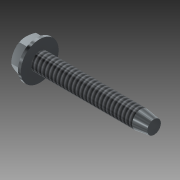
# Autodesk Inventor part: am-1266
Saved by Autodesk Inventor 2018 (Build 220112000, 112)
## iProperties
IsCustomPart: 0
Category: Screw Kit
Company: Autodesk Inc.
Created: 2017-12-13
Part Number: am-1266
Material: Steel, Mild
Description: Plain Indented Hex Washer Head Tapping Screw - Type C - Inch
Document SubType Name: Modeling
Standard: ANSI B18.6.4
Designer: Autodesk Inc.
Standard Revision: 1998
Standards Organization: ANSI
Language: en-US
Size Designation: 10-24 UNC - 1.25
Categories: <MemberInstance><Categories><Category DisplayName="Fasteners" InternalName="e4da775c-781d-43d5-af7c-5136215cf5a6" Mnemonic="FSTN"><Category DisplayName="Bolts" InternalName="536e6df0-f778-49ac-b2f2-25c71d2aa0b2" Mnemonic="SCRW"><CategoryParameter DisplayName="Nominal Diameter" InternalName="8bbe3f8e-44cf-40a9-a251-3a6edc8168d6" Mnemonic="nomdia"/><CategoryParameter DisplayName="Nominal Length" InternalName="238ecbaf-3e6c-45dd-aa95-4068c8e0fd02" Mnemonic="nomlen"/><CategoryParameter DisplayName="Thread Series Designation" InternalName="87c5849c-b3a5-4c3e-9c9b-2feecef9be86" Mnemonic="thrserdsgn"/><CategoryParameter DisplayName="Thread Class" InternalName="ebc0d23b-2cc6-4d2a-b376-d52aae53bab6" Mnemonic="thrclss"/><CategoryParameter DisplayName="Thread Designation" InternalName="586d5e89-370a-4089-914f-0110033585c7" Mnemonic="thrdesign"/><CategoryParameter DisplayName="Thread Type" InternalName="b4bbb7bc-d6aa-4c9f-a9a9-4152b9f6fe49" Mnemonic="thrtype"/><CategoryParameter DisplayName="Threads per Unit" InternalName="bdc6e7d2-ffd0-4d9c-a173-16b95ebb912d" Mnemonic="thrperunit1"/><CategoryParameter DisplayName="Thread Pitch" InternalName="bb82302e-82d8-4176-8fc1-c5d7bb17d5ad" Mnemonic="pitch1"/><CategoryParameter DisplayName="Nominal Diameter Designation" InternalName="03caf894-eafd-4c09-a035-916ac084b87b" Mnemonic="nomdiadesig"/><Category DisplayName="Hex Head - Flanged" InternalName="7925b6b6-1575-406f-8bfa-fe006e82b7bc" Mnemonic="FGPLSCREW"><CategoryParameter DisplayName="Shank Diameter" InternalName="6799ed14-8456-4cfb-bc01-ee9ecb2cdc2b" Mnemonic="grpdia"/><CategoryParameter DisplayName="Grip Length" InternalName="a82b65ac-2d41-4fd1-ba9a-aaa8c8b996d2" Mnemonic="grplen"/><CategoryParameter DisplayName="Thread Length" InternalName="f423544c-1850-46c6-9c68-3a3846636699" Mnemonic="thrlen"/><CategoryParameter DisplayName="Width Across Corners" InternalName="6c4712eb-409b-4c09-a24f-32eb670e2942" Mnemonic="wacor"/><CategoryParameter DisplayName="Head Height" InternalName="5df4f2f2-b824-4910-9115-49166ccd53b4" Mnemonic="headh"/><CategoryParameter DisplayName="Width Across Flats" InternalName="448f2cb5-f593-46ea-8e76-5090215a815d" Mnemonic="waflat"/><CategoryParameter DisplayName="Type" InternalName="851a99d2-714c-4be1-b4b1-e391fdc059ef" Mnemonic="type"/><Category DisplayName="Self Tapping Screws" InternalName="d7140fde-561b-401c-9855-a656e4b6870c" Mnemonic="FLPLCNRGTPSCRW"/></Category></Category></Category><Category DisplayName="DataType" InternalName="23b78d0f-2648-40c6-8793-ca6db495c9e8" Mnemonic="DATATYPE"><CategoryParameter DisplayName="DisplayName" InternalName="05415f3d-3907-474b-a020-eb9d644f4cf3" Mnemonic="DISPLAYNAME"/><CategoryParameter DisplayName="InternalName" InternalName="cf1d0246-76d9-4b4a-8305-fa0409afb5c1" Mnemonic="INTERNALNAME"/><CategoryParameter DisplayName="Folder Name" InternalName="3f06958e-8713-4116-9be7-ed6184ecc97b" Mnemonic="FOLDERNAME"/><CategoryParameter DisplayName="Family Version" InternalName="914462f6-6e19-4b14-ba84-155b9680b1d0" Mnemonic="FAMILYREVISION"/><CategoryParameter DisplayName="ClipFormat" InternalName="bc51e27b-3422-4e78-93ef-cec197ddf230" Mnemonic="CLIPFORMAT"/><CategoryParameter DisplayName="IsMetric" InternalName="e2385c5b-1ea4-4823-96a8-8de651266ec3" Mnemonic="ISMETRIC"/><CategoryParameter DisplayName="Description" InternalName="13903e3d-64b1-4950-80da-f627842ea37f" Mnemonic="DESCRIPTION"/><CategoryParameter DisplayName="StdsOrg" InternalName="8f5914e1-4693-403f-8ab5-d37768198c9d" Mnemonic="STDSORG"/><CategoryParameter DisplayName="Standard" InternalName="0c0a119c-1e12-4c84-803f-101930972f5e" Mnemonic="STANDARD"/><CategoryParameter DisplayName="Manufacturer" InternalName="cd6c7a72-a28a-4e50-99a9-2c7f4e13e5ad" Mnemonic="MANUFACTURER"/><CategoryParameter DisplayName="Member Revision" InternalName="a65d44b9-392f-4f4f-857b-e4b3d54996fe" Mnemonic="MEMBERREVISION"/><CategoryParameter DisplayName="Standard Revision" InternalName="91d5a463-65c2-4fde-b823-3b7fea5e8e17" Mnemonic="STANDARDREVISION"/><CategoryParameter DisplayName="Revision Guid" InternalName="45a75005-10b1-4dfc-8d6d-dfe629f0b93c" Mnemonic="REVISIONGUID"/><CategoryParameter DisplayName="Designation" InternalName="2675968c-4ce5-49e0-a4f5-552d29089031" Mnemonic="DESIGNATION"/><CategoryParameter DisplayName="FileName" InternalName="8b46a4cc-9585-4fed-90c3-899f57e09a73" Mnemonic="FILENAME"/><CategoryParameter DisplayName="Default Row" InternalName="2af9ec52-faaa-4026-b378-f9fa4afca842" Mnemonic="DEFAULTROW"/><Category DisplayName="Part" InternalName="c0e0b642-3bcb-4cc8-9e80-f96d35c4afa4" Mnemonic="PART"><CategoryParameter DisplayName="Material" InternalName="818a152a-d3c3-49ca-80ee-df7d91421b8e" Mnemonic="MATERIAL"/><CategoryParameter DisplayName="Material Key" InternalName="5c9a8adb-dd2b-4535-b97f-0a94a95fe41f" Mnemonic="MATERIALKEY"/><CategoryParameter DisplayName="Part Number" InternalName="016b6077-bfbe-49bd-92c9-d8d59c39c941" Mnemonic="PARTNUMBER"/><CategoryParameter DisplayName="Stock Number" InternalName="4dba7c1c-e26c-444e-836c-b08b433409a8" Mnemonic="STOCKNUMBER"/></Category></Category><Category DisplayName="LegacyMap" InternalName="cd87c42b-3e48-431e-b5c0-1cbeb14dfe77" Mnemonic="LEGACYMAP"><CategoryParameter DisplayName="CatalogName" InternalName="d99d1e27-aa94-4de2-af4c-c348882a6f4f" Mnemonic="CATALOGNAME"/><CategoryParameter DisplayName="FamilyNumber" InternalName="e705e1f4-09cb-413e-91f9-551b4188271e" Mnemonic="FAMILYNUMBER"/><CategoryParameter DisplayName="MemberID" InternalName="8e5e0294-fc51-4c8f-b3d7-003dc5ed94f6" Mnemonic="MEMBERID"/><CategoryParameter DisplayName="unique CC member ID" InternalName="5193edd4-b2b0-4ab4-9d54-de900eee34e0" Mnemonic="CCCOOKIE"/><CategoryParameter DisplayName="unique DA member ID" InternalName="0918ad47-427f-4fed-ae26-24c81c58f590" Mnemonic="DACOOKIE"/><CategoryParameter DisplayName="Merge11 ID" InternalName="0ee8fb18-e2ed-4f39-96f6-1f4b5f50aa71" Mnemonic="MERGE11"/><CategoryParameter DisplayName="Split ID" InternalName="72b5c83c-be7f-45c4-ae51-9160ea6deb26" Mnemonic="SPLIT"/></Category></Categories><FamilyTemplate Id="sh0007"><FamilyTemplateParameters><FamilyTemplateParameter ObjectType="kUserParameterObject" ValueType="xs:double" Id="1" ObjectReferenceKey="KOH"/><FamilyTemplateParameter ObjectType="kUserParameterObject" ValueType="xs:double" Id="2" ObjectReferenceKey="GD2"/><FamilyTemplateParameter ObjectType="kUserParameterObject" ValueType="xs:double" Id="3" ObjectReferenceKey="TPU"/><FamilyTemplateParameter ObjectType="kUserParameterObject" ValueType="xs:double" Id="4" ObjectReferenceKey="SD"/><FamilyTemplateParameter ObjectType="kUserParameterObject" ValueType="xs:double" Id="5" ObjectReferenceKey="GD1"/><FamilyTemplateParameter ObjectType="kUserParameterObject" ValueType="xs:double" Id="6" ObjectReferenceKey="GEL"/><FamilyTemplateParameter ObjectType="kUserParameterObject" ValueType="xs:double" Id="7" ObjectReferenceKey="SW"/><FamilyTemplateParameter ObjectType="kUserParameterObject" ValueType="xs:double" Id="8" ObjectReferenceKey="THREADDIA"/><FamilyTemplateParameter ObjectType="kUserParameterObject" ValueType="xs:double" Id="9" ObjectReferenceKey="TOA"/><FamilyTemplateParameter ObjectType="kUserParameterObject" ValueType="xs:double" Id="10" ObjectReferenceKey="NLG"/><FamilyTemplateParameter ObjectType="kUserParameterObject" ValueType="xs:double" Id="11" ObjectReferenceKey="PTC"/><FamilyTemplateParameter ObjectType="kUserParameterObject" ValueType="xs:double" Id="12" ObjectReferenceKey="NND"/><FamilyTemplateParameter ObjectType="kUserParameterObject" ValueType="xs:double" Id="13" ObjectReferenceKey="SB"/><FamilyTemplateParameter ObjectType="kUserParameterObject" ValueType="xs:double" Id="14" ObjectReferenceKey="SPTZ"/><FamilyTemplateParameter ObjectType="kUserParameterObject" ValueType="xs:double" Id="15" ObjectReferenceKey="SD3"/><FamilyTemplateParameter ObjectType="kUserParameterObject" ValueType="xs:double" Id="16" ObjectReferenceKey="SD2"/><FamilyTemplateParameter ObjectType="kUserParameterObject" ValueType="xs:double" Id="17" ObjectReferenceKey="E0"/><FamilyTemplateParameter ObjectType="kPropertyObject" ValueType="xs:string" Id="100" ObjectReferenceKey="{32853F0F-3444-11d1-9E93-0060B03C1CA6}" SubObjectId="52"/><FamilyTemplateParameter ObjectType="kPropertyObject" ValueType="xs:string" Id="105" ObjectReferenceKey="{32853F0F-3444-11d1-9E93-0060B03C1CA6}" SubObjectId="5"/><FamilyTemplateParameter ObjectType="kPartComponentDefinitionObject" ValueType="xs:string" Id="110" SubObjectId="Material"/><FamilyTemplateParameter ObjectType="kThreadFeatureObject" ValueType="xs:structure" Id="300" ObjectReferenceKey="1002000010000000ad200000000000008000000000000000" SubObjectId="ThreadInfo"><FamilyTemplateParameter ObjectType="" ValueType="xs:string" Id="301" SubObjectId="ThreadDesignation"/><FamilyTemplateParameter ObjectType="" ValueType="xs:string" Id="302" SubObjectId="ThreadType"/><FamilyTemplateParameter ObjectType="" ValueType="xs:string" Id="303" SubObjectId="ThreadClass"/></FamilyTemplateParameter></FamilyTemplateParameters></FamilyTemplate><CategoryParameterMap><ParamToTemplateMap><ParamToTemplate CategoryParameter="//CategoryParameter[@InternalName='05415f3d-3907-474b-a020-eb9d644f4cf3']" ConstantValue="Plain Indented Hex Washer Head Tapping Screw - Type C - Inch"/><ParamToTemplate CategoryParameter="//CategoryParameter[@InternalName='cf1d0246-76d9-4b4a-8305-fa0409afb5c1']" ConstantValue="d649e813-dc5c-4466-8ee0-86f1dc2aa72b"/><ParamToTemplate CategoryParameter="//CategoryParameter[@InternalName='3f06958e-8713-4116-9be7-ed6184ecc97b']" ConstantValue="ANSI B18.6.4(232)"/><ParamToTemplate CategoryParameter="//CategoryParameter[@InternalName='914462f6-6e19-4b14-ba84-155b9680b1d0']" ConstantValue="10"/><ParamToTemplate CategoryParameter="//CategoryParameter[@InternalName='bc51e27b-3422-4e78-93ef-cec197ddf230']" ConstantValue="CF_INVENTOR.STDPARTS"/><ParamToTemplate CategoryParameter="//CategoryParameter[@InternalName='e2385c5b-1ea4-4823-96a8-8de651266ec3']" ConstantValue="false"/><ParamToTemplate CategoryParameter="//CategoryParameter[@InternalName='13903e3d-64b1-4950-80da-f627842ea37f']" ConstantValue="Plain Indented Hex Washer Head Tapping Screw - Type C - Inch"/><ParamToTemplate CategoryParameter="//CategoryParameter[@InternalName='8f5914e1-4693-403f-8ab5-d37768198c9d']" ConstantValue="ANSI"/><ParamToTemplate CategoryParameter="//CategoryParameter[@InternalName='0c0a119c-1e12-4c84-803f-101930972f5e']" ConstantValue="ANSI B18.6.4"/><ParamToTemplate CategoryParameter="//CategoryParameter[@InternalName='cd6c7a72-a28a-4e50-99a9-2c7f4e13e5ad']" TemplateParameter="104"/><ParamToTemplate CategoryParameter="//CategoryParameter[@InternalName='91d5a463-65c2-4fde-b823-3b7fea5e8e17']" ConstantValue="1998"/><ParamToTemplate CategoryParameter="//CategoryParameter[@InternalName='45a75005-10b1-4dfc-8d6d-dfe629f0b93c']" ConstantValue="daae674b-f34b-45e6-9f46-31a5b4692541"/><ParamToTemplate CategoryParameter="//CategoryParameter[@InternalName='2af9ec52-faaa-4026-b378-f9fa4afca842']" ConstantValue="10"/><ParamToTemplate CategoryParameter="//CategoryParameter[@InternalName='d99d1e27-aa94-4de2-af4c-c348882a6f4f']" ConstantValue="ANSI"/><ParamToTemplate CategoryParameter="//CategoryParameter[@InternalName='e705e1f4-09cb-413e-91f9-551b4188271e']" ConstantValue="902"/><ParamToTemplate CategoryParameter="//CategoryParameter[@InternalName='8b46a4cc-9585-4fed-90c3-899f57e09a73']" ConstantValue="ANSI B18.6.4 - 10-24 UNC - 1.25(17) C"/><ParamToTemplate CategoryParameter="//CategoryParameter[@InternalName='a65d44b9-392f-4f4f-857b-e4b3d54996fe']" ConstantValue="4d9bfe0b-fef6-4d20-a557-dd97682ee487"/><ParamToTemplate CategoryParameter="//CategoryParameter[@InternalName='6799ed14-8456-4cfb-bc01-ee9ecb2cdc2b']" ConstantValue="0.19"/><ParamToTemplate CategoryParameter="//CategoryParameter[@InternalName='a82b65ac-2d41-4fd1-ba9a-aaa8c8b996d2']" ConstantValue="0"/><ParamToTemplate CategoryParameter="//CategoryParameter[@InternalName='5df4f2f2-b824-4910-9115-49166ccd53b4']" ConstantValue="0.151"/><ParamToTemplate CategoryParameter="//CategoryParameter[@InternalName='ebc0d23b-2cc6-4d2a-b376-d52aae53bab6']" ConstantValue="2A"/><ParamToTemplate CategoryParameter="//CategoryParameter[@InternalName='b4bbb7bc-d6aa-4c9f-a9a9-4152b9f6fe49']" ConstantValue="ANSI Unified Screw Threads"/><ParamToTemplate CategoryParameter="//CategoryParameter[@InternalName='8e5e0294-fc51-4c8f-b3d7-003dc5ed94f6']" ConstantValue="790"/><ParamToTemplate CategoryParameter="//CategoryParameter[@InternalName='2675968c-4ce5-49e0-a4f5-552d29089031']" TemplateParameter="100"/><ParamToTemplate CategoryParameter="//CategoryParameter[@InternalName='6c4712eb-409b-4c09-a24f-32eb670e2942']" TemplateParameter="17"/><ParamToTemplate CategoryParameter="//CategoryParameter[@InternalName='f423544c-1850-46c6-9c68-3a3846636699']" TemplateParameter="6"/><ParamToTemplate CategoryParameter="//CategoryParameter[@InternalName='818a152a-d3c3-49ca-80ee-df7d91421b8e']" TemplateParameter="110"/><ParamToTemplate CategoryParameter="//CategoryParameter[@InternalName='238ecbaf-3e6c-45dd-aa95-4068c8e0fd02']" TemplateParameter="10"/><ParamToTemplate CategoryParameter="//CategoryParameter[@InternalName='8bbe3f8e-44cf-40a9-a251-3a6edc8168d6']" TemplateParameter="12"/><ParamToTemplate CategoryParameter="//CategoryParameter[@InternalName='016b6077-bfbe-49bd-92c9-d8d59c39c941']" TemplateParameter="105"/><ParamToTemplate CategoryParameter="//CategoryParameter[@InternalName='bb82302e-82d8-4176-8fc1-c5d7bb17d5ad']" TemplateParameter="11"/><ParamToTemplate CategoryParameter="//CategoryParameter[@InternalName='586d5e89-370a-4089-914f-0110033585c7']" TemplateParameter="301"/><ParamToTemplate CategoryParameter="//CategoryParameter[@InternalName='bdc6e7d2-ffd0-4d9c-a173-16b95ebb912d']" TemplateParameter="3"/></ParamToTemplateMap></CategoryParameterMap></MemberInstance>
Density: 1 g/cm^3
Catalog Web Link: http://www.andymark.com/Search-s/545.htm?Search=10-32+x+0.5&Submit=
Vendor: AndyMark Inc.
Appearance: Zinc
Author: Autodesk Inc.
Keywords: Drive Base Kit
Autodesk Inventor part; units mm, degrees
ref_plane "YZ Plane" through (0, 0, 0) normal (1, 0, 0) x (0, 1, 0)
sketch "Sketch1" plane through (0, 0, 0) normal (0, 0, 1) x (1, 0, 0)
  line L0 (-0.7874, 5.2578) -> (-0.7874, 0)
  line L1 (-0.7874, 0) -> (31.75, 0)
  line L2 (31.75, 0) -> (31.75, 2.413)
  line L3 (31.75, 2.413) -> (0, 2.413)
  line L4 (0, 2.413) -> (0, 5.2578)
  line L5 (-7.2949, 0) -> (38.2575, 0) projected
  line L6 (0, -1.0516) -> (0, 6.3094) projected
  line L7 (0, 5.2578) -> (-0.7874, 5.2578)
  dimension "d1" = 0.7874
  dimension "d2" = 4.826
  dimension "d3" = 31.75
  dimension "d22" = 10.5156
  constraints: 12 end point, 4 perpendicular, 2 collinear, 1 point on line, 1 vertical
  measures "d1" distance between parallel lines of L0 L4
  measures "d2" diameter of L3 L1
  measures "d3" distance between parallel lines of L2 L4
  measures "d22" diameter of L7 L1
revolve "Body" add sketch "Sketch1" angle 360 about axis through (-0.7874, 0, 0) along (1, 0, 0)
sketch "Sketch2" plane through (-0.7874, 0, 0) normal (-1, 0, 0) x (0, 0, 1)
  line L0 (0, 4.5754) -> (3.9624, 2.2877)
  line L1 (3.9624, 2.2877) -> (3.9624, -2.2877)
  line L2 (3.9624, -2.2877) -> (0, -4.5754)
  line L3 (0, -4.5754) -> (-3.9624, -2.2877)
  line L4 (-3.9624, -2.2877) -> (-3.9624, 2.2877)
  line L5 (-3.9624, 2.2877) -> (0, 4.5754)
  circle A0 centre (0, 0) radius 5.2578 projected
  dimension "d11" = 7.9248
  constraints: 12 end point, 1 coincident, 1 vertical, 11 other
  measures "d11" distance between parallel lines of L1 L4
extrude "Head" add sketch "Sketch2" along normal blind 3.048 contours L0 L1 L2 L3 L4 L5
ref_plane "IDS_WORKPLANE{1}" through (-3.8354, 0, 0) normal (-1, 0, 0) x (0, 0, -1)
sketch "Sketch3" plane through (-3.8354, 0, 0) normal (-1, 0, 0) x (0, 0, -1)
  circle A0 centre (0, 0) radius 3.1699
  point P0 (0, 0)
  dimension "d15" = 6.3398
  constraints: 1 centre point, 1 coincident
  measures "d15" diameter of A0
extrude "Indent" cut sketch "Sketch3" against normal blind 0.3048
thread "Thread" size "10-24 UNC" class "2A" standard "ANSI Unified Screw Threads" length 31.75
sketch "Sketch4" plane through (0, 0, 0) normal (0, 0, 1) x (1, 0, 0)
  line L0 (-3.8354, 3.9624) -> (-3.8354, 4.5754)
  line L1 (-3.8354, 4.5754) -> (-3.3472, 4.5754)
  line L2 (-3.8354, 4.5754) -> (-3.8354, 2.2877) projected
  line L3 (-4.9666, 0) -> (2.8908, 0) projected
  line L4 (-0.7874, 4.5754) -> (-3.8354, 4.5754) projected
  arc A0 (-3.3472, 4.5754) -> (-3.8354, 3.9624) centre (1.7683, 0) ccw
  dimension "d21" = 7.9248
  dimension "d23" = 6.8631
  constraints: 4 end point, 2 collinear, 2 point on circle, 2 point on line, 1 centre point, 1 perpendicular, 1 vertical
  measures "d21" diameter of L0.start L3
  measures "d23" radius of A0
revolve "Chamfer1" cut sketch "Sketch4" angle 360 about axis through (-10, 0, 0) along (1, 0, 0)
chamfer "Chamfer2" distance 0.5334 distance2 3.7084 1 edges at (31.75, -2.413, 0) measured on face at (31.75, 0.5787, 0.3409)
ref_plane "Work Plane3" through (7, 0, 0) normal (0, 0, -1) x (1, 0, 0)
equation "\"d1\" = SD"
equation "\"d2\" = NND"
equation "\"d3\" = NLG"
equation "\"d22\" = SD2"
equation "\"d11\" = SW"
equation "\"d12\" = KOH"
equation "\"d15\" = SD3"
equation "\"d16\" = SB"
equation "\"d21\" = SW"
equation "\"d23\" = 0.866025 * SW"
equation "\"d6\" = GEL"
equation "\"d19\" = -0.5 * GD2 + 0.5 * NND"
equation "\"d20\" = SPTZ"
equation "\"NLG\" = 31.75"
equation "\"NND\" = 4.826"
equation "\"KOH\" = 3.048"
equation "\"GEL\" = 31.75"
equation "\"SW\" = 7.9248"
equation "\"GD2\" = 3.7592"
equation "\"SPTZ\" = 3.7084"
equation "\"SD3\" = 0.8 * SW"
equation "\"SB\" = 0.1 * KOH"
equation "\"SD2\" = 10.5156"
equation "\"SD\" = 0.7874"
equation "\"GD1\" = 3.7592"
equation "\"THREADDIA\" = 4.826"
equation "\"TOA\" = 30deg"
equation "\"E0\" = 9.15077"
body "Solid1"
